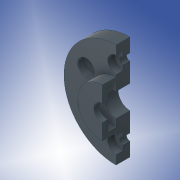
# Autodesk Inventor part: BA008
Saved by Autodesk Inventor 2017 SP1 (Build 210196100, 196)
## iProperties
Created: 2017-06-15
Part Number: BA008
Material: ABS Plastic
Document SubType Name: Modeling
Designer: zallen
Density: 1.06 g/cm^3
Appearance: CR Dark Blue
Author: zallen
Autodesk Inventor part; units mm, degrees
ref_plane "YZ Plane" through (0, 0, 0) normal (1, 0, 0) x (0, 1, 0)
ref_plane "XZ Plane" through (0, 0, 0) normal (0, 1, 0) x (-1, 0, 0)
ref_plane "XY Plane" through (0, 0, 0) normal (0, 0, 1) x (1, 0, 0)
sketch "Sketch1" plane through (0, 0, 0) normal (0, 0, 1) x (1, 0, 0)
  circle A0 centre (0, 0) radius 37.5
  circle A1 centre (0, 25) radius 2.5
  circle A2 centre (0, 0) radius 25 construction
  circle A3 centre (-21.6506, 12.5) radius 2.5
  circle A4 centre (-21.6506, -12.5) radius 2.5
  circle A5 centre (0, -25) radius 2.5
  circle A6 centre (21.6506, -12.5) radius 2.5
  circle A7 centre (21.6506, 12.5) radius 2.5
  circle A8 centre (0, 0) radius 2.5
  dimension "d2" = 50
  dimension "d0" = 75
  dimension "d1" = 5
  dimension "d5" = 360
  dimension "d7" = 5
  constraints: 8 centre point, 3 coincident, 2 vertical alignment, 15 other
  measures "d0" diameter of A0
  measures "d1" diameter of A1
  measures "d7" diameter of A8
extrude "Extrusion1" add sketch "Sketch1" along normal blind 10
sketch "Sketch4" plane through (0, 0, 10) normal (0, 0, 1) x (1, 0, 0)
  circle A0 centre (0, 0) radius 2.5 projected
  circle A1 centre (21.6506, 12.5) radius 2.5 projected
  circle A2 centre (21.6506, -12.5) radius 2.5 projected
  circle A3 centre (0, -25) radius 2.5 projected
  circle A4 centre (-21.6506, -12.5) radius 2.5 projected
  circle A5 centre (-21.6506, 12.5) radius 2.5 projected
  circle A6 centre (0, 25) radius 2.5 projected
  circle A7 centre (0, 0) radius 37.5 projected
  circle A8 centre (0, 25) radius 6
  circle A9 centre (-21.6506, 12.5) radius 6
  circle A10 centre (-21.6506, -12.5) radius 6
  circle A11 centre (0, -25) radius 6
  circle A12 centre (21.6506, -12.5) radius 6
  circle A13 centre (21.6506, 12.5) radius 6
  dimension "d17" = 12
  dimension "d20" = 360
  constraints: 6 centre point, 6 coincident, 19 other
  measures "d17" diameter of A8
extrude "Extrusion4" cut sketch "Sketch4" against normal blind 5 contours A8 | A9 | A10 | A11 | A12 | A13
sketch "Sketch5" plane through (0, 0, 0) normal (0, 0, -1) x (-1, 0, 0)
  circle A0 centre (0, 0) radius 2.5 projected
  circle A1 centre (0, 0) radius 8.5
  dimension "d24" = 17
  constraints: 1 centre point, 1 coincident
  measures "d24" diameter of A1
extrude "Extrusion5" cut sketch "Sketch5" against normal blind 5
sketch "Sketch6" plane through (0, 0, 10) normal (0, 0, 1) x (1, 0, 0)
  circle A0 centre (0, 0) radius 2.5 projected
  circle A1 centre (0, 0) radius 14
  circle A2 centre (0, 0) radius 17.5
  dimension "d35" = 35
  dimension "d36" = 28
  constraints: 2 centre point, 1 coincident
  measures "d35" diameter of A2
  measures "d36" diameter of A1
extrude "Extrusion6" add sketch "Sketch6" along normal blind 10 contours A2
sketch "Sketch7" plane through (0, 0, 20) normal (0, 0, 1) x (1, 0, 0)
  circle A0 centre (0, 0) radius 6
  circle A1 centre (0, 0) radius 2.5
  circle A2 centre (0, 0) radius 17.5
  circle A3 centre (0, 0) radius 17.5 projected
  dimension "d40" = 12
  constraints: 3 centre point, 2 coincident, 1 concentric
  measures "d40" diameter of A0
extrude "Extrusion7" add sketch "Sketch7" against normal blind 4 contours A2
sketch "Sketch8" plane through (0, 0, 20) normal (0, 0, 1) x (1, 0, 0)
  circle A0 centre (0, 0) radius 37.5 projected
  line L0 (0, -37.5) -> (37.5, -37.5)
  line L1 (37.5, -37.5) -> (37.5, 37.5)
  line L2 (37.5, 37.5) -> (0, 37.5)
  line L3 (0, 37.5) -> (0, -37.5)
  point P0 (37.5, 0)
  constraints: 8 end point, 2 midpoint, 2 parallel, 2 point on circle, 1 coincident, 1 horizontal, 1 perpendicular
extrude "Extrusion8" cut sketch "Sketch8" against normal through all contours A0 L3 | L1 L0 A0 | A0 L2 L1 picked at (9.7729, 7.7936)
sketch "Sketch9" plane through (0, 0, 5) normal (0, 0, -1) x (-1, 0, 0)
  arc A0 (0, 14) -> (0, -14) centre (0, 0) ccw projected
  circle A1 centre (0, 0) radius 8.5 construction
  arc A2 (0, -14) -> (0, 14) centre (0, 0) ccw projected
  line L0 (0, 14) -> (-0.0015, 8.5)
  line L1 (0, -14) -> (0, -8.5)
  line L2 (0, -6) -> (0, -14) projected
  arc A3 (0, -8.5) -> (-0.0015, 8.5) centre (0, 0) ccw
  line L3 (0, 8.5) -> (0, 2.5) projected
  dimension "d39" = 17
  constraints: 4 end point, 4 point on circle, 3 centre point, 1 coincident, 1 concentric, 1 point on line
  measures "d39" diameter of A1
extrude "Extrusion9" cut sketch "Sketch9" against normal blind 5 contours L0 A3 L1 A0
body "Solid1"
